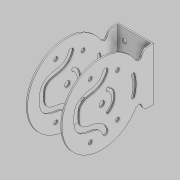
# Autodesk Inventor part: RR-PCSS-2021-W2M2MA-kopia
Saved by Autodesk Inventor 2021 (Build 250183000, 183)
## iProperties
Created: 2021-09-01
Part Number: RR-PCSS-2021-W2M2MA-kopia
Material: Ogólny
Document SubType Name: Konstrukcja blachowa
Designer: marci
Density: 1 g/cm^3
Sheet Metal Rule: Domyślny_mm
Appearance: Domyślna
Author: marci
Autodesk Inventor part; units mm, degrees
ref_plane "YZ Plane" through (0, 0, 0) normal (1, 0, 0) x (0, 1, 0)
ref_plane "XZ Plane" through (0, 0, 0) normal (0, 1, 0) x (-1, 0, 0)
ref_plane "XY Plane" through (0, 0, 0) normal (0, 0, 1) x (1, 0, 0)
sketch "Szkic1" plane through (0, 0, 0) normal (1, 0, 0) x (0, 1, 0)
  circle A0 centre (113.6112, 151.2877) radius 4.15
  spline S0 degree 3 poles (74.022, 83.1836) (74.0852, 84.0135) (74.2951, 84.8221) (75.0094, 86.4279) (75.5325, 87.1921) (77.3483, 89.1263) (78.76, 89.913) (80.7709, 90.8615) (81.5783, 91.1764) (82.2628, 91.4986) knots -0.848671 -0.848671 -0.848671 -0.848671 -0.699684 -0.699684 -0.534513 -0.534513 -0.226958 -0.226958 -0.000001 -0.000001 -0.000001 -0.000001
  line L0 (74.022, 83.1836) -> (74.0852, 84.0135) construction
  line L1 (74.0852, 84.0135) -> (74.2951, 84.8221) construction
  line L2 (74.2951, 84.8221) -> (75.0094, 86.4279) construction
  line L3 (75.0094, 86.4279) -> (75.5325, 87.1921) construction
  line L4 (75.5325, 87.1921) -> (77.3483, 89.1263) construction
  line L5 (77.3483, 89.1263) -> (78.76, 89.913) construction
  line L6 (78.76, 89.913) -> (80.7709, 90.8615) construction
  line L7 (80.7709, 90.8615) -> (81.5783, 91.1764) construction
  line L8 (81.5783, 91.1764) -> (82.2628, 91.4986) construction
  spline S1 degree 3 poles (73.5762, 72.7639) (73.6109, 75.6361) (73.7134, 78.5183) (73.9342, 81.9795) (73.9762, 82.5813) (74.022, 83.1836) knots -1.663427 -1.663427 -1.663427 -1.663427 -0.802776 -0.802776 -0.622027 -0.622027 -0.622027 -0.622027
  line L9 (73.5762, 72.7639) -> (73.6109, 75.6361) construction
  line L10 (73.6109, 75.6361) -> (73.7134, 78.5183) construction
  line L11 (73.7134, 78.5183) -> (73.9342, 81.9795) construction
  line L12 (73.9342, 81.9795) -> (73.9762, 82.5813) construction
  line L13 (73.9762, 82.5813) -> (74.022, 83.1836) construction
  line L14 (153.6461, 72.7639) -> (73.5762, 72.7639)
  spline S2 degree 3 poles (153.2003, 83.1836) (153.2598, 82.401) (153.3129, 81.6191) (153.5215, 78.1565) (153.6136, 75.4566) (153.6461, 72.7639) knots -1.042689 -1.042689 -1.042689 -1.042689 -0.807866 -0.807866 0 0 0 0
  line L15 (153.2003, 83.1836) -> (153.2598, 82.401) construction
  line L16 (153.2598, 82.401) -> (153.3129, 81.6191) construction
  line L17 (153.3129, 81.6191) -> (153.5215, 78.1565) construction
  line L18 (153.5215, 78.1565) -> (153.6136, 75.4566) construction
  line L19 (153.6136, 75.4566) -> (153.6461, 72.7639) construction
  spline S3 degree 3 poles (144.9596, 91.4986) (145.498, 91.2451) (146.0735, 91.0122) (147.8651, 90.2182) (149.2392, 89.5381) (151.462, 87.5517) (152.0498, 86.6611) (152.8529, 85.0872) (153.1258, 84.1506) (153.1993, 83.1827) knots -0.979854 -0.979854 -0.979854 -0.979854 -0.818823 -0.818823 -0.528853 -0.528853 -0.291221 -0.291221 -0.000001 -0.000001 -0.000001 -0.000001
  line L20 (144.9596, 91.4986) -> (145.498, 91.2451) construction
  line L21 (145.498, 91.2451) -> (146.0735, 91.0122) construction
  line L22 (146.0735, 91.0122) -> (147.8651, 90.2182) construction
  line L23 (147.8651, 90.2182) -> (149.2392, 89.5381) construction
  line L24 (149.2392, 89.5381) -> (151.462, 87.5517) construction
  line L25 (151.462, 87.5517) -> (152.0498, 86.6611) construction
  line L26 (152.0498, 86.6611) -> (152.8529, 85.0872) construction
  line L27 (152.8529, 85.0872) -> (153.1258, 84.1506) construction
  line L28 (153.1258, 84.1506) -> (153.1993, 83.1827) construction
  spline S4 degree 3 poles (142.9599, 93.0001) (143.125, 92.7763) (143.3181, 92.5751) (143.9503, 92.0303) (144.4527, 91.7372) (144.9595, 91.4985) knots 0 0 0 0 0.333229 0.333229 1 1 1 1
  line L29 (142.9599, 93.0001) -> (143.125, 92.7763) construction
  line L30 (143.125, 92.7763) -> (143.3181, 92.5751) construction
  line L31 (143.3181, 92.5751) -> (143.9503, 92.0303) construction
  line L32 (143.9503, 92.0303) -> (144.4527, 91.7372) construction
  line L33 (144.4527, 91.7372) -> (144.9595, 91.4985) construction
  spline S5 degree 3 poles (142.0824, 95.0135) (142.1143, 94.8561) (142.1534, 94.7002) (142.3639, 93.9985) (142.622, 93.4585) (142.9599, 93.0001) knots 0 0 0 0 0.21917 0.21917 1 1 1 1
  line L34 (142.0824, 95.0135) -> (142.1143, 94.8561) construction
  line L35 (142.1143, 94.8561) -> (142.1534, 94.7002) construction
  line L36 (142.1534, 94.7002) -> (142.3639, 93.9985) construction
  line L37 (142.3639, 93.9985) -> (142.622, 93.4585) construction
  line L38 (142.622, 93.4585) -> (142.9599, 93.0001) construction
  line L39 (144.3569, 99.7639) -> (142.0824, 95.0135)
  arc A1 (144.3569, 99.7639) -> (82.8655, 99.7639) centre (113.6112, 151.2877) ccw
  line L40 (85.14, 95.0135) -> (82.8655, 99.7639)
  spline S6 degree 3 poles (84.2624, 93.0001) (84.4744, 93.2875) (84.6534, 93.6051) (84.9484, 94.2773) (85.0651, 94.6428) (85.1402, 95.0135) knots 0 0 0 0 0.487768 0.487768 1 1 1 1
  line L41 (84.2624, 93.0001) -> (84.4744, 93.2875) construction
  line L42 (84.4744, 93.2875) -> (84.6534, 93.6051) construction
  line L43 (84.6534, 93.6051) -> (84.9484, 94.2773) construction
  line L44 (84.9484, 94.2773) -> (85.0651, 94.6428) construction
  line L45 (85.0651, 94.6428) -> (85.1402, 95.0135) construction
  spline S7 degree 3 poles (82.2628, 91.4986) (82.5199, 91.6196) (82.7648, 91.7494) (83.4026, 92.1387) (83.791, 92.4382) (84.1596, 92.8659) (84.2125, 92.9321) (84.2626, 93) knots 0 0 0 0 0.322742 0.322742 0.897788 0.897788 1 1 1 1
  line L46 (82.2628, 91.4986) -> (82.5199, 91.6196) construction
  line L47 (82.5199, 91.6196) -> (82.7648, 91.7494) construction
  line L48 (82.7648, 91.7494) -> (83.4026, 92.1387) construction
  line L49 (83.4026, 92.1387) -> (83.791, 92.4382) construction
  line L50 (83.791, 92.4382) -> (84.1596, 92.8659) construction
  line L51 (84.1596, 92.8659) -> (84.2125, 92.9321) construction
  line L52 (84.2125, 92.9321) -> (84.2626, 93) construction
  spline S8 degree 3 poles (154.8329, 149.6931) (153.2858, 150.1946) (151.7715, 150.8339) (149.173, 152.3598) (148.074, 153.1859) (145.5424, 155.7112) (144.4219, 157.4993) (141.8184, 163.751) (141.4067, 168.6628) (139.6953, 176.9058) (138.8143, 179.6863) (135.9855, 184.6966) (134.3085, 186.8287) (130.6294, 190.0144) (128.6311, 191.2234) (122.4331, 193.2437) (118.3111, 193.4955) (113.6112, 193.4955) knots -9.163844 -9.163844 -9.163844 -9.163844 -8.462986 -8.462986 -7.866788 -7.866788 -6.925416 -6.925416 -4.962347 -4.962347 -3.570014 -3.570014 -2.417257 -2.417257 -1.409976 -1.409976 0 0 0 0
  line L53 (154.8329, 149.6931) -> (153.2858, 150.1946) construction
  line L54 (153.2858, 150.1946) -> (151.7715, 150.8339) construction
  line L55 (151.7715, 150.8339) -> (149.173, 152.3598) construction
  line L56 (149.173, 152.3598) -> (148.074, 153.1859) construction
  line L57 (148.074, 153.1859) -> (145.5424, 155.7112) construction
  line L58 (145.5424, 155.7112) -> (144.4219, 157.4993) construction
  line L59 (144.4219, 157.4993) -> (141.8184, 163.751) construction
  line L60 (141.8184, 163.751) -> (141.4067, 168.6628) construction
  line L61 (141.4067, 168.6628) -> (139.6953, 176.9058) construction
  line L62 (139.6953, 176.9058) -> (138.8143, 179.6863) construction
  line L63 (138.8143, 179.6863) -> (135.9855, 184.6966) construction
  line L64 (135.9855, 184.6966) -> (134.3085, 186.8287) construction
  line L65 (134.3085, 186.8287) -> (130.6294, 190.0144) construction
  line L66 (130.6294, 190.0144) -> (128.6311, 191.2234) construction
  line L67 (128.6311, 191.2234) -> (122.4331, 193.2437) construction
  line L68 (122.4331, 193.2437) -> (118.3111, 193.4955) construction
  line L69 (118.3111, 193.4955) -> (113.6112, 193.4955) construction
  arc A2 (152.3658, 142.083) -> (154.8329, 149.6931) centre (153.5994, 145.8881) ccw
  spline S9 degree 3 poles (113.6112, 185.4955) (117.8973, 185.4955) (121.1661, 185.2621) (125.0168, 183.9758) (126.1008, 183.3655) (128.7031, 181.081) (129.9478, 179.2928) (132.7795, 173.461) (133.0932, 167.8083) (135.0085, 159.5209) (135.9039, 156.6602) (139.2342, 150.5668) (141.3916, 148.442) (146.0388, 144.5107) (149.5071, 143.0098) (152.3658, 142.083) knots -3.192679 -3.192679 -3.192679 -3.192679 -2.821868 -2.821868 -2.622552 -2.622552 -2.337236 -2.337236 -1.651686 -1.651686 -1.313895 -1.313895 -0.901553 -0.901553 0 0 0 0
  line L70 (113.6112, 185.4955) -> (117.8973, 185.4955) construction
  line L71 (117.8973, 185.4955) -> (121.1661, 185.2621) construction
  line L72 (121.1661, 185.2621) -> (125.0168, 183.9758) construction
  line L73 (125.0168, 183.9758) -> (126.1008, 183.3655) construction
  line L74 (126.1008, 183.3655) -> (128.7031, 181.081) construction
  line L75 (128.7031, 181.081) -> (129.9478, 179.2928) construction
  line L76 (129.9478, 179.2928) -> (132.7795, 173.461) construction
  line L77 (132.7795, 173.461) -> (133.0932, 167.8083) construction
  line L78 (133.0932, 167.8083) -> (135.0085, 159.5209) construction
  line L79 (135.0085, 159.5209) -> (135.9039, 156.6602) construction
  line L80 (135.9039, 156.6602) -> (139.2342, 150.5668) construction
  line L81 (139.2342, 150.5668) -> (141.3916, 148.442) construction
  line L82 (141.3916, 148.442) -> (146.0388, 144.5107) construction
  line L83 (146.0388, 144.5107) -> (149.5071, 143.0098) construction
  line L84 (149.5071, 143.0098) -> (152.3658, 142.083) construction
  spline S10 degree 3 poles (74.8565, 142.083) (76.5982, 142.6476) (78.7085, 143.4772) (82.6164, 145.7582) (84.2399, 146.9811) (88.3904, 151.0764) (89.9814, 153.9667) (93.1671, 161.5054) (93.6608, 167.0043) (95.2462, 174.7896) (95.9193, 176.7023) (97.7584, 179.9865) (98.8711, 181.4057) (101.1497, 183.3765) (102.228, 183.9959) (106.1422, 185.2674) (109.3742, 185.4955) (113.6112, 185.4955) knots -6.764215 -6.764215 -6.764215 -6.764215 -6.337153 -6.337153 -5.984104 -5.984104 -5.327189 -5.327189 -3.865631 -3.865631 -2.879053 -2.879053 -1.999784 -1.999784 -1.271086 -1.271086 0 0 0 0
  line L85 (74.8565, 142.083) -> (76.5982, 142.6476) construction
  line L86 (76.5982, 142.6476) -> (78.7085, 143.4772) construction
  line L87 (78.7085, 143.4772) -> (82.6164, 145.7582) construction
  line L88 (82.6164, 145.7582) -> (84.2399, 146.9811) construction
  line L89 (84.2399, 146.9811) -> (88.3904, 151.0764) construction
  line L90 (88.3904, 151.0764) -> (89.9814, 153.9667) construction
  line L91 (89.9814, 153.9667) -> (93.1671, 161.5054) construction
  line L92 (93.1671, 161.5054) -> (93.6608, 167.0043) construction
  line L93 (93.6608, 167.0043) -> (95.2462, 174.7896) construction
  line L94 (95.2462, 174.7896) -> (95.9193, 176.7023) construction
  line L95 (95.9193, 176.7023) -> (97.7584, 179.9865) construction
  line L96 (97.7584, 179.9865) -> (98.8711, 181.4057) construction
  line L97 (98.8711, 181.4057) -> (101.1497, 183.3765) construction
  line L98 (101.1497, 183.3765) -> (102.228, 183.9959) construction
  line L99 (102.228, 183.9959) -> (106.1422, 185.2674) construction
  line L100 (106.1422, 185.2674) -> (109.3742, 185.4955) construction
  line L101 (109.3742, 185.4955) -> (113.6112, 185.4955) construction
  arc A3 (72.3895, 149.6931) -> (74.8565, 142.083) centre (73.623, 145.8881) ccw
  spline S11 degree 3 poles (113.6112, 193.4955) (108.9529, 193.4955) (104.8625, 193.2481) (98.6696, 191.2626) (96.675, 190.0647) (92.7038, 186.6731) (90.7949, 184.1356) (86.6312, 175.9278) (86.3428, 169.6779) (84.56, 161.9198) (83.8799, 159.7321) (81.8564, 156.0282) (80.6818, 154.5636) (77.4787, 151.8565) (75.2736, 150.6281) (72.3895, 149.6931) knots -7.999364 -7.999364 -7.999364 -7.999364 -6.854457 -6.854457 -6.025354 -6.025354 -4.914124 -4.914124 -2.60919 -2.60919 -1.693088 -1.693088 -0.909563 -0.909563 0 0 0 0
  line L102 (113.6112, 193.4955) -> (108.9529, 193.4955) construction
  line L103 (108.9529, 193.4955) -> (104.8625, 193.2481) construction
  line L104 (104.8625, 193.2481) -> (98.6696, 191.2626) construction
  line L105 (98.6696, 191.2626) -> (96.675, 190.0647) construction
  line L106 (96.675, 190.0647) -> (92.7038, 186.6731) construction
  line L107 (92.7038, 186.6731) -> (90.7949, 184.1356) construction
  line L108 (90.7949, 184.1356) -> (86.6312, 175.9278) construction
  line L109 (86.6312, 175.9278) -> (86.3428, 169.6779) construction
  line L110 (86.3428, 169.6779) -> (84.56, 161.9198) construction
  line L111 (84.56, 161.9198) -> (83.8799, 159.7321) construction
  line L112 (83.8799, 159.7321) -> (81.8564, 156.0282) construction
  line L113 (81.8564, 156.0282) -> (80.6818, 154.5636) construction
  line L114 (80.6818, 154.5636) -> (77.4787, 151.8565) construction
  line L115 (77.4787, 151.8565) -> (75.2736, 150.6281) construction
  line L116 (75.2736, 150.6281) -> (72.3895, 149.6931) construction
  arc A4 (98.6112, 101.4981) -> (128.6112, 101.4981) centre (113.6112, 151.2877) ccw
  arc A5 (100.0535, 106.2856) -> (98.6112, 101.4981) centre (99.3323, 103.8919) ccw
  arc A6 (100.0535, 106.2856) -> (127.1689, 106.2856) centre (113.6112, 151.2877) ccw
  arc A7 (128.6112, 101.4981) -> (127.1689, 106.2856) centre (127.89, 103.8919) ccw
  circle A8 centre (81.2505, 127.7763) radius 3.65
  circle A9 centre (72.1885, 168.8706) radius 3.65
  circle A10 centre (155.0339, 168.8706) radius 3.65
  circle A11 centre (145.9719, 127.7763) radius 3.65
  arc A12 (100.7634, 143.546) -> (126.459, 143.546) centre (113.6112, 151.2877) ccw
  arc A13 (130.7416, 140.9654) -> (126.459, 143.546) centre (128.6003, 142.2557) ccw
  arc A14 (96.4808, 140.9654) -> (130.7416, 140.9654) centre (113.6112, 151.2877) ccw
  arc A15 (100.7634, 143.546) -> (96.4808, 140.9654) centre (98.6221, 142.2557) ccw
  point P0 (0, 0)
  point P1 (144.9591, 91.4987)
  point P2 (85.1399, 95.0119)
  point P3 (84.2622, 92.9995)
  point P4 (100.7634, 143.546)
  point P5 (100.0535, 106.2856)
  point P6 (152.3658, 142.083)
  point P7 (113.611, 185.4955)
  point P8 (113.6106, 193.4955)
  dimension "d0" = 7.3
  dimension "d1" = 4
  dimension "d2" = 2.5
  dimension "d3" = 60
  dimension "d4" = 52
  dimension "d5" = 20
  dimension "d6" = 8.3
  dimension "d7" = 71.347
  dimension "d8" = 70.084
  dimension "d9" = 68.591
  dimension "d10" = 68.155
  dimension "d11" = 67.691
  dimension "d12" = 67.692
  dimension "d13" = 55.798
  dimension "d14" = 175.076
  dimension "d15" = 45.004
  dimension "d16" = 38.613
  dimension "d17" = 167.538
  dimension "d18" = 23.824
  dimension "d19" = 161.032
  dimension "d20" = 8.371
  dimension "d21" = 5.439
  dimension "d22" = 5.94
  dimension "d23" = 153.033
  dimension "d24" = 4.073
  dimension "d25" = 7.256
  dimension "d26" = 140.033
  dimension "d27" = 12.296
  dimension "d28" = 22.268
  dimension "d29" = 22.791
  dimension "d30" = 28.211
  dimension "d31" = 82.376
  dimension "d32" = 130.571
  dimension "d33" = 35.639
  dimension "d34" = 46.493
  dimension "d35" = 55.345
  dimension "d36" = 57.925
  dimension "d37" = 60.596
  dimension "d38" = 112.753
  dimension "d39" = 119.691
  dimension "d40" = 26.603
  dimension "d41" = 125.543
  dimension "d42" = 43.38
  dimension "d43" = 42.59
  dimension "d44" = 125.341
  dimension "d45" = 33.851
  dimension "d46" = 120.975
  dimension "d47" = 111.138
  dimension "d48" = 22.927
  dimension "d49" = 133.861
  dimension "d50" = 13.213
  dimension "d51" = 142.802
  dimension "d52" = 23.317
  dimension "d53" = 11.415
  dimension "d54" = 0.092
  dimension "d55" = 0.51
  dimension "d56" = 14.467
  dimension "d57" = 13.879
  dimension "d58" = 17.962
  dimension "d59" = 21.997
  dimension "d60" = 21.422
  dimension "d61" = 35.957
  dimension "d62" = 35.738
  dimension "d63" = 47.839
  constraints: 22 point on circle, 16 centre point, 10 tangent, 9 parallel, 7 equal radius, 6 end point, 4 concentric, 1 coincident, 1 collinear, 1 perpendicular, 36 other
  measures "d0" diameter of A10
  measures "d1" radius of A2
  measures "d2" radius of A13
  measures "d3" radius of A1
  measures "d4" radius of A4
  measures "d5" radius of A14
  measures "d6" diameter of A0
  measures "d7" angle of L19 L53
  measures "d8" angle of L18 L53
  measures "d9" angle of L17 L53
  measures "d10" angle of L16 L53
  measures "d11" angle of L15 L53
  measures "d12" angle of L28 L53
  measures "d13" angle of L27 L53
  measures "d14" angle of L54 L53
  measures "d15" angle of L26 L53
  measures "d16" angle of L25 L53
  measures "d17" angle of L55 L53
  measures "d18" angle of L24 L53
  measures "d19" angle of L56 L53
  measures "d20" angle of L23 L53
  measures "d21" angle of L53 L83
  measures "d22" angle of L22 L53
  measures "d23" angle of L57 L53
  measures "d24" angle of L21 L53
  measures "d25" angle of L20 L53
  measures "d26" angle of L53 L58
  measures "d27" angle of L32 L53
  measures "d28" angle of L53 L82
  measures "d29" angle of L31 L53
  measures "d30" angle of L30 L53
  measures "d31" angle of L39 L53
  measures "d32" angle of L53 L59
  measures "d33" angle of L29 L53
  measures "d34" angle of L37 L53
  measures "d35" angle of L36 L53
  measures "d36" angle of L35 L53
  measures "d37" angle of L34 L53
  measures "d38" angle of L53 L60
  measures "d39" angle of L53 L61
  measures "d40" angle of L53 L81
  measures "d41" angle of L53 L62
  measures "d42" angle of L53 L80
  measures "d43" angle of L53 L63
  measures "d44" angle of L53 L79
  measures "d45" angle of L53 L64
  measures "d46" angle of L53 L78
  measures "d47" angle of L53 L77
  measures "d48" angle of L53 L65
  measures "d49" angle of L53 L76
  measures "d50" angle of L53 L66
  measures "d51" angle of L53 L75
  measures "d52" angle of L53 L74
  measures "d53" angle of L53 L73
  measures "d54" angle of L53 L67
  measures "d55" angle of L53 L72
  measures "d56" angle of L53 L68
  measures "d57" angle of L53 L71
  measures "d58" angle of L53 L69
  measures "d59" angle of L53 L100
  measures "d60" angle of L53 L103
  measures "d61" angle of L53 L99
  measures "d62" angle of L53 L104
  measures "d63" angle of L53 L98
extrude "Wyciągnięcie proste1" add sketch "Szkic1" along normal blind 2
sketch "Szkic2" plane through (2, 0, 0) normal (1, 0, 0) x (0, 0, -1)
  line L0 (-74.7639, 73.5762) -> (-74.7639, 153.6461)
  line L1 (-72.7639, 73.5762) -> (-72.7639, 153.6461) projected
  ellipse E0 centre (-19.9458, 118.0537) end of major axis (-124.6183, 93.4754) minor radius 38.0945 (-83.1836, 74.022) -> (-72.7639, 73.5762) ccw projected
  ellipse E1 centre (-28.9439, 115.9985) end of major axis (-122.9992, 134.9118) minor radius 33.2195 (-72.7639, 153.6461) -> (-83.1827, 153.1999) ccw projected
  point P0 (0, 0)
  point P1 (-74.7639, 153.6109)
  point P2 (-74.7639, 73.6114)
  dimension "d295" = 2
  constraints: 2 end point, 1 vertical, 2 other
  measures "d295" distance between parallel lines of L1 L0
extrude "Wyciągnięcie proste2" add sketch "Szkic2" along normal blind 50
ref_plane "Płaszczyzna konstrukcyjna1" through (27, 0, 0) normal (1, 0, 0) x (0, 0, -1)
mirror "Odbij1" about plane through (27, 0, 0) normal (1, 0, 0) of "Wyciągnięcie proste1"
sketch "Szkic4" plane through (0, 0, 0) normal (-1, 0, 0) x (0, 0, 1)
  circle A0 centre (127.7763, 81.2505) radius 3.65 projected
  circle A1 centre (127.7763, 81.2505) radius 3
  circle A2 centre (168.8706, 72.1885) radius 3.65 projected
  circle A3 centre (168.8706, 72.1885) radius 3
  circle A4 centre (168.8706, 155.0339) radius 3.65 projected
  circle A5 centre (168.8706, 155.0339) radius 3
  circle A6 centre (127.7763, 145.9719) radius 3.65 projected
  circle A7 centre (127.7763, 145.9719) radius 3
  circle A8 centre (127.7763, 145.9719) radius 3.65 projected
  circle A9 centre (168.8706, 155.0339) radius 3.65 projected
  point P0 (0, 0)
  dimension "d305" = 6
  dimension "d306" = 6
  dimension "d307" = 6
  dimension "d308" = 6
  constraints: 4 centre point, 4 coincident
  measures "d305" diameter of A1
  measures "d306" diameter of A3
  measures "d307" diameter of A5
  measures "d308" diameter of A7
extrude "Wyciągnięcie proste4" add sketch "Szkic4" against normal up to surface (2 mm away)
mirror "Odbij3" about plane through (27, 0, 0) normal (1, 0, 0) of "Wyciągnięcie proste4"
sketch "Szkic5" plane through (0, 73.5762, 72.7639) normal (0, 0, -1) x (-1, 0, 0)
  line L0 (0, 25.035) -> (0, 55.035) projected
  line L1 (0, 40.035) -> (-62.5062, 40.035)
  point P0 (0, -73.5762)
  constraints: 2 end point, 1 horizontal, 1 midpoint
ref_plane "Płaszczyzna konstrukcyjna2" through (0, 113.6112, 72.7639) normal (0, 1, 0) x (1, 0, 0)
sketch "Szkic6" plane through (2, 73.6114, 74.7639) normal (0, 0, 1) x (1, 0, 0)
  point P0 (10, 16.9997)
  point P1 (10, 62.9997)
  point P2 (42, 62.9997)
  point P3 (42, 16.9997)
hole "Otwór1" at (12, 90.6112, 74.7639) at (12, 136.6112, 74.7639) at (44, 136.6112, 74.7639) at (44, 90.6112, 74.7639) direction (0, 0, -1) diameter 6.6 end through all
equation "\"PromieńGięcia\" = Grubość"
equation "\"SzerokośćGięciaPodcięcia\" = Grubość"
equation "\"GłębokośćGięciaPodcięcia\" = 0.5 * Grubość"
equation "\"RozmiarPodcięciaNarożnika\" = 4 * Grubość"
equation "\"MinimalnaPozostałość\" = 2 * Grubość"
equation "\"PromieńPrzejścia\" = PromieńGięcia"
equation "\"Rozmiar_promienia_Jacobiego\" = PromieńGięcia"
equation "\"Wielk_odstępu\" = Grubość"
equation "\"Grubość\" = 0.5"
